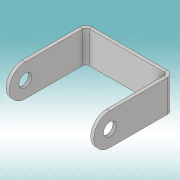
# Autodesk Inventor part: SHEET_METAL1
Saved by Autodesk Inventor 2019 (Build 230136000, 136)
## iProperties
Created: 2019-02-05
Part Number: SHEET_METAL1
Material: Generic
Document SubType Name: Sheet Metal
Designer: nelson.soberon
Density: 1 g/cm^3
Sheet Metal Rule: Default_mm
Appearance: Default
Author: nelson.soberon
Autodesk Inventor part; units mm, degrees
ref_plane "YZ Plane" through (0, 0, 0) normal (1, 0, 0) x (0, 1, 0)
ref_plane "XZ Plane" through (0, 0, 0) normal (0, 1, 0) x (-1, 0, 0)
ref_plane "XY Plane" through (0, 0, 0) normal (0, 0, 1) x (1, 0, 0)
sketch "Sketch1" plane through (0, 0, 0) normal (0, 0, 1) x (1, 0, 0)
  line L0 (0, 0) -> (27.5, 0)
  line L1 (27.5, -20) -> (0, -20)
  line L2 (0, 0) -> (0, -20)
  line L3 (0, 0) -> (-27.5, 0)
  line L4 (-27.5, -20) -> (0, -20)
  line L5 (27.5, 0) -> (27.5, -20)
  line L6 (-27.5, 0) -> (-27.5, -20)
  dimension "d0" = 27.5
  dimension "d6" = 20
  constraints: 14 end point, 2 horizontal, 2 symmetric about line, 2 vertical, 1 parallel
  measures "d0" distance of L0.start L0.end
  measures "d6" distance of L0.end L1.start
extrude "Extrusion1" add sketch "Sketch1" along normal mid plane 2
sketch "Sketch2" plane through (-25.5, -20, -1) normal (-1, 0, 0) x (0, -1, 0)
  line L0 (-20, 0) -> (0, 0)
  line L1 (0, 0) -> (0, 50)
  line L2 (0, 50) -> (-20, 50)
  line L3 (-20, 50) -> (-20, 0)
  constraints: 6 end point, 1 horizontal, 1 perpendicular, 1 vertical
edge flange "Flange1" height 50 angle 90 thickness 2 bend radius 2 thickness toward (-1, 0, 0) relief tear relief width 2 relief depth 1 edges at (-27.5, -10, 1) wall of the first edge with corners at (-25.5, 0, -1) (-25.5, -20, -1) (-25.5, -20, 49) (-25.5, 0, 49)
bend "Bend1"
corner "Corner1"
sketch "Sketch3" plane through (25.5, 0, -1) normal (1, 0, 0) x (0, 1, 0)
  line L0 (-20, 0) -> (0, 0)
  line L1 (0, 0) -> (0, 50)
  line L2 (0, 50) -> (-20, 50)
  line L3 (-20, 50) -> (-20, 0)
  constraints: 6 end point, 1 horizontal, 1 perpendicular, 1 vertical
edge flange "Flange2" height 50 angle 90 thickness 2 bend radius 2 thickness toward (1, 0, 0) relief tear relief width 2 relief depth 1 edges at (27.5, -10, 1) wall of the first edge with corners at (25.5, -20, -1) (25.5, 0, -1) (25.5, 0, 49) (25.5, -20, 49)
bend "Bend2"
corner "Corner2"
sketch "Sketch5" plane through (27.5, -20, 49) normal (1, 0, 0) x (0, 0, -1)
  line L0 (46, 0) -> (0, 0) projected
  line L1 (0, 0) -> (0, 20) projected
  line L2 (0, 20) -> (0, 0) projected
  line L3 (0, 0) -> (0, 20)
  line L4 (0, 20) -> (10, 20)
  line L5 (0, 0) -> (10, 0)
  line L6 (0, 0) -> (46, 0) projected
  arc A0 (10, 20) -> (10, 0) centre (10, 10) ccw
  line L7 (0, 20) -> (46, 20) projected
  circle A1 centre (10, 10) radius 4
  point P0 (49, 20)
  point P1 (0, 10)
  dimension "d38" = 10
  dimension "d39" = 10
  dimension "d40" = 10
  dimension "d46" = 8
  constraints: 6 end point, 3 coincident, 3 point on circle, 2 centre point, 2 point on line
  measures "d38" distance of L0.end L5.end
  measures "d39" distance of L1.end L4.end
  measures "d40" radius of A0
  measures "d46" diameter of A1
extrude "Cut1" cut sketch "Sketch5" against normal blind 2
sketch "Sketch6" plane through (-27.5, -20, 49) normal (-1, 0, 0) x (0, 0, 1)
  line L0 (0, 20) -> (0, 0) projected
  line L1 (-10, 0) -> (0, 0)
  line L2 (0, 0) -> (0, 20)
  line L3 (0, 20) -> (-10, 20)
  line L4 (-46, 20) -> (0, 20) projected
  arc A0 (-10, 0) -> (-10, 20) centre (-10, 10) ccw
  circle A1 centre (-10, 10) radius 4
  point P0 (-49, 20)
  point P1 (0, 10)
  dimension "d43" = 10
  dimension "d47" = 8
  constraints: 6 end point, 3 coincident, 3 point on circle, 2 centre point, 1 midpoint, 1 perpendicular, 1 point on line
  measures "d43" distance of L1.start L0.end
  measures "d47" diameter of A1
extrude "Cut2" cut sketch "Sketch6" against normal blind 2
sketch "Sketch7" plane through (0, 0, -1) normal (0, 0, -1) x (-1, 0, 0)
  line L0 (23.5, 0) -> (-23.5, 0) projected
  line L1 (-23.5, -20) -> (23.5, -20) projected
  circle A0 centre (0, -10) radius 4.5
  line L2 (23.5, -20) -> (23.5, 0) projected
  line L3 (-23.5, 0) -> (-23.5, -20) projected
  point P0 (0, 0)
  dimension "d48" = 10
  dimension "d49" = 9
  dimension "d53" = 23.5
  constraints: 1 centre point
  measures "d48" distance from line of L0 A0.centre
  measures "d49" diameter of A0
  measures "d53" distance from line of A0.centre L2
extrude "Extrusion2" add sketch "Sketch7" along normal blind 0.1 contours A0
equation "\"d41\" = Thickness"
equation "\"d44\" = Thickness"
equation "\"d7\" = Thickness"
equation "\"d8\" = BendReliefWidth"
equation "\"d9\" = BendReliefDepth"
equation "\"d10\" = MinimumRemnant"
equation "\"d11\" = TransitionRadius"
equation "\"d14\" = BendRadius"
equation "\"d15\" = CornerReliefSize"
equation "\"d16\" = GapSize"
equation "\"d17\" = JacobiRadiusSize"
equation "\"d18\" = BendReliefWidth"
equation "\"d19\" = BendReliefDepth"
equation "\"d20\" = MinimumRemnant"
equation "\"d21\" = TransitionRadius"
equation "\"d24\" = BendRadius"
equation "\"d25\" = CornerReliefSize"
equation "\"d26\" = GapSize"
equation "\"d27\" = JacobiRadiusSize"
equation "\"BendRadius\" = Thickness"
equation "\"BendReliefWidth\" = Thickness"
equation "\"BendReliefDepth\" = 0.5 * Thickness"
equation "\"CornerReliefSize\" = 4 * Thickness"
equation "\"MinimumRemnant\" = 2 * Thickness"
equation "\"TransitionRadius\" = BendRadius"
equation "\"JacobiRadiusSize\" = BendRadius"
equation "\"GapSize\" = Thickness"
equation "\"Thickness\" = 2"
body "Solid1"
